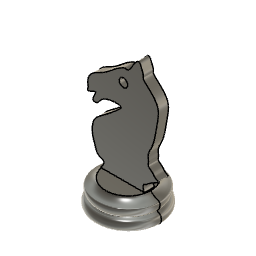
knight (Autodesk Fusion 360 design; units mm, degrees)
Autodesk Fusion 360 part; units mm, degrees
sketch "Sketch1" plane through (0, 0, 0) normal (0, 1, 0) x (1, 0, 0) in component "knight"
  line L0 (0, 0) -> (15, 0) construction
  line L1 (15, 0) -> (15, -50) construction
  line L2 (15, -50) -> (0, -50) construction
  line L3 (0, -50) -> (0, 0) construction
  spline S0 degree 5 poles (0, 0) (0.0526, -0.0012) (0.1627, -0.0035) (0.3425, -0.0061) (0.6115, -0.008) (0.996, -0.0079) (1.4274, -0.0055) (1.9028, -0.0012) (2.4173, 0.0043) (2.9632, 0.0101) (3.5309, 0.0147) (4.1102, 0.0172) (4.6902, 0.0165) (5.2615, 0.012) (5.8161, 0.004) (6.3488, -0.0066) (6.8581, -0.0178) (7.346, -0.0267) (7.8165, -0.0302) (8.2751, -0.0262) (8.7271, -0.0134) (9.177, 0.0074) (9.6271, 0.033) (10.0772, 0.0573) (10.5247, 0.0721) (10.9648, 0.068) (11.3906, 0.0347) (11.7937, -0.0382) (12.1638, -0.1606) (12.4896, -0.341) (12.761, -0.5841) (12.9698, -0.8897) (13.1112, -1.2507) (13.1861, -1.6509) (13.1992, -2.0678) (13.1574, -2.4766) (13.0671, -2.8546) (12.9331, -3.1847) (12.7551, -3.4605) (12.5306, -3.6857) (12.2623, -3.8696) (11.9643, -4.0228) (11.6697, -4.1531) (11.4344, -4.2623) (11.3133, -4.3545) (11.3409, -4.4418) (11.5045, -4.5545) (11.7552, -4.7313) (12.0312, -5.0035) (12.2772, -5.3812) (12.4643, -5.8402) (12.5817, -6.3358) (12.6312, -6.8147) (12.6209, -7.2274) (12.5593, -7.5401) (12.4484, -7.7489) (12.2813, -7.8829) (12.0507, -7.9841) (11.7539, -8.0939) (11.4001, -8.2348) (11.0078, -8.4134) (10.6006, -8.6253) (10.2039, -8.8594) (9.8412, -9.1022) (9.53, -9.3428) (9.2804, -9.5749) (9.1341, -9.7513) (9.0551, -9.8779) (9.0161, -9.9597) (9, -10) knots 0 0 0 0 0 0 0.01538462 0.03076923 0.04615385 0.06153846 0.07692308 0.09230769 0.10769231 0.12307692 0.13846154 0.15384615 0.16923077 0.18461538 0.2 0.21538462 0.23076923 0.24615385 0.26153846 0.27692308 0.29230769 0.30769231 0.32307692 0.33846154 0.35384615 0.36923077 0.38461538 0.4 0.41538462 0.43076923 0.44615385 0.46153846 0.47692308 0.49230769 0.50769231 0.52307692 0.53846154 0.55384615 0.56923077 0.58461538 0.6 0.61538462 0.63076923 0.64615385 0.66153846 0.67692308 0.69230769 0.70769231 0.72307692 0.73846154 0.75384615 0.76923077 0.78461538 0.8 0.81538462 0.83076923 0.84615385 0.86153846 0.87692308 0.89230769 0.90769231 0.92307692 0.93846154 0.95384615 0.96923077 0.98461538 1 1 1 1 1 1
  line L4 (9, -10) -> (0, -10)
  line L5 (0, -10) -> (0, 0)
  point P0 (2, 0)
  point P1 (6, 0)
  point P2 (9, 0)
  point P3 (11.5484, 0)
  point P4 (13, -1)
  point P5 (13, -3)
  point P6 (12, -4)
  point P7 (11.3429, -4.3777)
  point P8 (12, -5)
  point P9 (12.5759, -7.4088)
  point P10 (12, -8)
  point P11 (10, -9)
  dimension "d1" = 15
  dimension "d2" = 50
  constraint horizontal L0
  constraint vertical L1
  constraint horizontal L2
  constraint vertical L3
  constraint coincident L0.start L3.end
  constraint coincident L3 L4.end
  constraint perpendicular L3 L4
  measures "d1" distance of L0.start L0.end
  measures "d2" distance of L0.start L2.end
revolve "Revolve1" add sketch "Sketch1" angle 360 about axis through (0, 0, 50) along (0, 0, -1) in component "knight"
sketch "Sketch2" plane through (0, 0, 0) normal (0, 1, 0) x (1, 0, 0) in component "knight"
  spline S0 degree 5 poles (9, -10) (8.9254, -9.9671) (8.7825, -9.9218) (8.587, -9.9156) (8.3643, -10.0307) (8.1495, -10.3671) (8.0001, -10.857) (7.9194, -11.4202) (7.911, -11.9582) (7.9755, -12.3843) (8.1097, -12.6474) (8.3024, -12.7683) (8.5364, -12.8373) (8.7965, -12.947) (9.0782, -13.131) (9.3827, -13.3759) (9.7105, -13.6467) (10.0537, -13.9111) (10.3945, -14.154) (10.7173, -14.3718) (11.0159, -14.5705) (11.3065, -14.7622) (11.6273, -14.9624) (12.013, -15.1841) (12.4772, -15.4337) (12.9868, -15.7055) (13.4542, -15.9793) (13.779, -16.2323) (13.8815, -16.4476) (13.7397, -16.6242) (13.4227, -16.7859) (13.0378, -16.9643) (12.6847, -17.1849) (12.401, -17.449) (12.1766, -17.7415) (11.9765, -18.0406) (11.7618, -18.3281) (11.5087, -18.5973) (11.2092, -18.8498) (10.8733, -19.0935) (10.532, -19.3398) (10.2334, -19.6008) (10.0214, -19.8849) (9.9222, -20.194) (9.9215, -20.5174) (9.9736, -20.8382) (10.0271, -21.144) (10.0485, -21.44) (10.0323, -21.7486) (9.9888, -22.0949) (9.9382, -22.4936) (9.9036, -22.941) (9.9078, -23.4243) (9.9692, -23.9277) (10.0986, -24.4389) (10.2948, -24.9571) (10.5472, -25.4904) (10.8392, -26.0526) (11.1512, -26.6599) (11.464, -27.3275) (11.7617, -28.0668) (12.0356, -28.8817) (12.2833, -29.7688) (12.5072, -30.7191) (12.7125, -31.7197) (12.9057, -32.7549) (13.0933, -33.808) (13.2793, -34.8621) (13.4646, -35.9024) (13.6446, -36.9167) (13.8076, -37.8978) (13.9343, -38.8437) (14.0009, -39.7564) (13.9828, -40.6404) (13.8569, -41.5012) (13.6052, -42.3444) (13.2179, -43.1737) (12.6964, -43.99) (12.0559, -44.7897) (11.3302, -45.5636) (10.5681, -46.2972) (9.8249, -46.9747) (9.1563, -47.5817) (8.6105, -48.108) (8.2211, -48.5503) (8, -48.9158) (7.9309, -49.2241) (7.9586, -49.5124) (8.0071, -49.8232) (8.0081, -50.1873) (7.9321, -50.6026) (7.792, -51.0366) (7.62, -51.4506) (7.4525, -51.8162) (7.3091, -52.1406) (7.1848, -52.4674) (7.0606, -52.837) (6.9098, -53.2621) (6.7066, -53.6859) (6.4307, -53.9985) (6.0695, -54.086) (5.6219, -53.8674) (5.1014, -53.3415) (4.5325, -52.5709) (3.9454, -51.6589) (3.372, -50.7295) (2.8411, -49.9055) (2.3738, -49.2876) (1.9789, -48.9333) (1.6485, -48.8356) (1.3531, -48.9023) (1.0568, -49.0079) (0.7304, -49.0425) (0.3684, -48.9688) (-0.0188, -48.8043) (-0.415, -48.5904) (-0.8087, -48.3658) (-1.2022, -48.1391) (-1.6068, -47.9001) (-2.0383, -47.6278) (-2.5125, -47.3002) (-3.0403, -46.9038) (-3.6242, -46.4404) (-4.2607, -45.9222) (-4.9412, -45.3692) (-5.6541, -44.8051) (-6.3858, -44.2544) (-7.1222, -43.7388) (-7.8503, -43.2741) (-8.56, -42.8661) (-9.2445, -42.509) (-9.8995, -42.1891) (-10.5224, -41.8872) (-11.1113, -41.5821) (-11.6641, -41.2531) (-12.1777, -40.8831) (-12.6468, -40.4618) (-13.0642, -39.9875) (-13.4215, -39.4657) (-13.7111, -38.9083) (-13.9274, -38.3329) (-14.0675, -37.7614) (-14.1333, -37.2201) (-14.1325, -36.7357) (-14.0801, -36.3263) (-13.9998, -35.9933) (-13.9258, -35.7135) (-13.9046, -35.4295) (-13.9654, -35.089) (-14.0943, -34.6791) (-14.1965, -34.2748) (-14.1447, -33.9927) (-13.8395, -33.9305) (-13.2816, -34.0987) (-12.5666, -34.4204) (-11.8361, -34.7748) (-11.2422, -35.0266) (-10.9067, -35.0607) (-10.8809, -34.8163) (-11.1109, -34.3168) (-11.4784, -33.6419) (-11.8359, -32.9037) (-12.0459, -32.2209) (-12.0132, -31.6957) (-11.7326, -31.3838) (-11.2814, -31.2916) (-10.7662, -31.3952) (-10.2846, -31.6532) (-9.8733, -32.0244) (-9.5139, -32.4702) (-9.1556, -32.9551) (-8.7317, -33.447) (-8.1797, -33.9181) (-7.4583, -34.3448) (-6.5692, -34.7091) (-5.5514, -34.9974) (-4.4693, -35.201) (-3.4025, -35.3149) (-2.4352, -35.3376) (-1.646, -35.2709) (-1.0964, -35.119) (-0.8219, -34.8886) (-0.8181, -34.5878) (-1.0439, -34.2263) (-1.441, -33.8145) (-1.9478, -33.3627) (-2.5177, -32.8813) (-3.1192, -32.3797) (-3.7329, -31.8669) (-4.3485, -31.3509) (-4.9625, -30.8387) (-5.5752, -30.3361) (-6.1882, -29.8476) (-6.8014, -29.3763) (-7.4114, -28.9237) (-8.0124, -28.4895) (-8.5972, -28.0714) (-9.1579, -27.6654) (-9.6864, -27.265) (-10.1756, -26.8617) (-10.6198, -26.4443) (-11.0158, -25.9995) (-11.3614, -25.5144) (-11.6555, -24.978) (-11.8977, -24.3832) (-12.0875, -23.7287) (-12.2241, -23.0217) (-12.306, -22.2773) (-12.3325, -21.5155) (-12.3039, -20.7579) (-12.2226, -20.0255) (-12.0937, -19.3351) (-11.926, -18.6967) (-11.7328, -18.1102) (-11.531, -17.5654) (-11.3366, -17.048) (-11.1614, -16.5435) (-11.009, -16.0421) (-10.8712, -15.5431) (-10.7241, -15.0603) (-10.536, -14.615) (-10.2782, -14.2287) (-9.9331, -13.9156) (-9.5053, -13.6747) (-9.0274, -13.4849) (-8.5483, -13.3132) (-8.1246, -13.1213) (-7.8114, -12.8712) (-7.6513, -12.5337) (-7.672, -12.0899) (-7.8903, -11.528) (-8.2298, -10.9796) (-8.5784, -10.5118) (-8.8525, -10.1748) (-9, -10) knots 0 0 0 0 0 0 0.00434783 0.00869565 0.01304348 0.0173913 0.02173913 0.02608696 0.03043478 0.03478261 0.03913043 0.04347826 0.04782609 0.05217391 0.05652174 0.06086957 0.06521739 0.06956522 0.07391304 0.07826087 0.0826087 0.08695652 0.09130435 0.09565217 0.1 0.10434783 0.10869565 0.11304348 0.1173913 0.12173913 0.12608696 0.13043478 0.13478261 0.13913043 0.14347826 0.14782609 0.15217391 0.15652174 0.16086957 0.16521739 0.16956522 0.17391304 0.17826087 0.1826087 0.18695652 0.19130435 0.19565217 0.2 0.20434783 0.20869565 0.21304348 0.2173913 0.22173913 0.22608696 0.23043478 0.23478261 0.23913043 0.24347826 0.24782609 0.25217391 0.25652174 0.26086957 0.26521739 0.26956522 0.27391304 0.27826087 0.2826087 0.28695652 0.29130435 0.29565217 0.3 0.30434783 0.30869565 0.31304348 0.3173913 0.32173913 0.32608696 0.33043478 0.33478261 0.33913043 0.34347826 0.34782609 0.35217391 0.35652174 0.36086957 0.36521739 0.36956522 0.37391304 0.37826087 0.3826087 0.38695652 0.39130435 0.39565217 0.4 0.40434783 0.40869565 0.41304348 0.4173913 0.42173913 0.42608696 0.43043478 0.43478261 0.43913043 0.44347826 0.44782609 0.45217391 0.45652174 0.46086957 0.46521739 0.46956522 0.47391304 0.47826087 0.4826087 0.48695652 0.49130435 0.49565217 0.5 0.50434783 0.50869565 0.51304348 0.5173913 0.52173913 0.52608696 0.53043478 0.53478261 0.53913043 0.54347826 0.54782609 0.55217391 0.55652174 0.56086957 0.56521739 0.56956522 0.57391304 0.57826087 0.5826087 0.58695652 0.59130435 0.59565217 0.6 0.60434783 0.60869565 0.61304348 0.6173913 0.62173913 0.62608696 0.63043478 0.63478261 0.63913043 0.64347826 0.64782609 0.65217391 0.65652174 0.66086957 0.66521739 0.66956522 0.67391304 0.67826087 0.6826087 0.68695652 0.69130435 0.69565217 0.7 0.70434783 0.70869565 0.71304348 0.7173913 0.72173913 0.72608696 0.73043478 0.73478261 0.73913043 0.74347826 0.74782609 0.75217391 0.75652174 0.76086957 0.76521739 0.76956522 0.77391304 0.77826087 0.7826087 0.78695652 0.79130435 0.79565217 0.8 0.80434783 0.80869565 0.81304348 0.8173913 0.82173913 0.82608696 0.83043478 0.83478261 0.83913043 0.84347826 0.84782609 0.85217391 0.85652174 0.86086957 0.86521739 0.86956522 0.87391304 0.87826087 0.8826087 0.88695652 0.89130435 0.89565217 0.9 0.90434783 0.90869565 0.91304348 0.9173913 0.92173913 0.92608696 0.93043478 0.93478261 0.93913043 0.94347826 0.94782609 0.95217391 0.95652174 0.96086957 0.96521739 0.96956522 0.97391304 0.97826087 0.9826087 0.98695652 0.99130435 0.99565217 1 1 1 1 1 1
  line L0 (-9, -10) -> (9, -10)
  circle A0 centre (0.1105, -43.6972) radius 1.6778
  point P0 (8.143, -10.4588)
  point P1 (8.0702, -12.5337)
  point P2 (8.5798, -12.8614)
  point P3 (9.5991, -13.553)
  point P4 (10.9096, -14.4995)
  point P5 (12.3657, -15.3731)
  point P6 (13.8217, -16.4288)
  point P7 (13, -17)
  point P8 (12, -18)
  point P9 (11, -19)
  point P10 (10, -20)
  point P11 (10, -21)
  point P12 (10, -22)
  point P13 (10, -24)
  point P14 (11.5359, -27.5236)
  point P15 (13.5987, -36.667)
  point P16 (12.4279, -44.3051)
  point P17 (8, -49)
  point P18 (8, -50)
  point P19 (7.5217, -51.6645)
  point P20 (7, -53)
  point P21 (6, -54)
  point P22 (2, -49)
  point P23 (1, -49)
  point P24 (-0.3952, -48.5981)
  point P25 (-2.4023, -47.3715)
  point P26 (-7.6431, -43.4131)
  point P27 (-12, -41)
  point P28 (-14, -38)
  point P29 (-14, -36)
  point P30 (-14, -35)
  point P31 (-14, -34)
  point P32 (-11, -35)
  point P33 (-12, -32)
  point P34 (-10.6537, -31.482)
  point P35 (-8, -34)
  point P36 (-1, -35)
  point P37 (-1.566, -33.7121)
  point P38 (-6, -30)
  point P39 (-10, -27)
  point P40 (-12, -24)
  point P41 (-12, -19)
  point P42 (-11, -16)
  point P43 (-10, -14)
  point P44 (-8, -13)
  constraint horizontal L0
extrude "Extrude1" add sketch "Sketch2" along normal mid plane 4 contours S0 L0 picked at (-2.7969, -19.9788) in component "knight"
component "knight" placed x (1, 0, 0) y (0, 1, 0) z (0, 0, 1) at (0, 0, 0)
